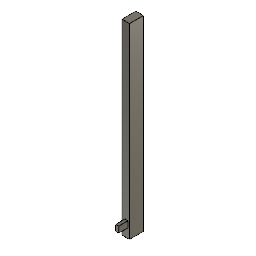
Arm Wheel Dowel Stop (Autodesk Fusion 360 design; units mm, degrees)
Autodesk Fusion 360 part; units mm, degrees
sketch "Sketch1" plane through (0, 0, 0) normal (0, 0, 1) x (1, 0, 0)
  line L0 (0, 0) -> (2.5, 0)
  line L1 (2.5, 0) -> (2.5, -4.5)
  line L2 (2.5, -4.5) -> (0, -4.5)
  line L3 (0, -4.5) -> (0, 0)
  dimension "d8" = 2.5
  dimension "d9" = 4.5
  constraint horizontal L0
  constraint vertical L1
  constraint horizontal L2
  constraint vertical L3
  constraint coincident L0.start L3.end
  measures "d8" distance of L0.start L0.end
  measures "d9" distance of L0.start L2.end
extrude "Extrude1" add sketch "Sketch1" along normal blind 60
sketch "Sketch2" plane through (0, -4.5, 0) normal (0, -1, 0) x (1, 0, 0)
  line L0 (0, 0) -> (2.5, 0)
  line L1 (2.5, 0) -> (2.5, 60)
  line L2 (2.5, 60) -> (0, 60)
  line L3 (0, 60) -> (0, 0)
  line L4 (1, 3) -> (2, 3)
  line L5 (2, 3) -> (2, 5)
  line L6 (2, 5) -> (1, 5)
  line L7 (1, 5) -> (1, 3)
  dimension "d12" = 1
  dimension "d13" = 2
  dimension "d16" = 3
  constraint horizontal L4
  constraint vertical L5
  constraint horizontal L6
  constraint vertical L7
  measures "d12" distance of L4.start L4.end
  measures "d13" distance of L4.start L6.end
  measures "d16" distance of L0 L4
extrude "Extrude2" add sketch "Sketch2" along normal blind 3 contours L4 L5 L6 L7
equation "length = 60 mm"
equation "width = 4.5 mm"
equation "height = 2.5 mm"
equation "dent_length = 3 mm"
equation "dent_width = 2 mm"
equation "dent_height = 1 mm"
equation "dent_distance = 3 mm"
equation "d8 = height"
equation "d9 = width"
equation "d10 = length"
equation "d12 = dent_height"
equation "d13 = dent_width"
equation "d14 = dent_length"
equation "d16 = dent_distance"
